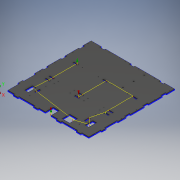
# Autodesk Inventor part: BA09
Saved by Autodesk Inventor 2017 (Build 210142000, 142)
## iProperties
Created: 2019-05-29
Part Number: BA09
Material: Wood (Cherry)
Document SubType Name: Modeling
Designer: Dell
Density: 0.63 g/cm^3
Appearance: Smooth - Black
Mass: 1071.87 g
Surface Area: 5591.98 cm^2
Volume: 1701.39 cm^3
Author: Dell
Autodesk Inventor part; units mm, degrees
(part 1 of 2)
ref_plane "YZ Plane" through (0, 0, 0) normal (1, 0, 0) x (0, 1, 0)
ref_plane "XZ Plane" through (0, 0, 0) normal (0, 1, 0) x (-1, 0, 0)
ref_plane "XY Plane" through (0, 0, 0) normal (0, 0, 1) x (1, 0, 0)
sketch "Sketch1" plane through (0, 0, 0) normal (0, 0, 1) x (1, 0, 0)
  line L0 (0, 0) -> (525.78, 0)
  line L1 (525.78, 0) -> (525.78, 355.6)
  line L2 (525.78, 355.6) -> (0, 355.6)
  line L3 (0, 355.6) -> (0, 0)
  dimension "d0" = 525.78
  dimension "d1" = 355.6
  constraints: 8 end point, 2 parallel, 1 horizontal, 1 perpendicular
  measures "d0" distance of L2.end L1.end
  measures "d1" distance of L2.end L0.start
extrude "Extrusion1" add sketch "Sketch1" along normal blind 6.35
sketch "Sketch2" plane through (0, 0, 6.35) normal (0, 0, 1) x (1, 0, 0)
  line L0 (525.78, 0) -> (525.78, 355.6) projected
  line L1 (525.78, 306.07) -> (518.16, 306.07)
  line L2 (518.16, 306.07) -> (518.16, 278.13)
  line L3 (518.16, 278.13) -> (525.78, 278.13)
  line L4 (525.78, 278.13) -> (525.78, 306.07)
  line L5 (525.78, 191.77) -> (518.16, 191.77)
  line L6 (518.16, 191.77) -> (518.16, 163.83)
  line L7 (518.16, 163.83) -> (525.78, 163.83)
  line L8 (525.78, 163.83) -> (525.78, 191.77)
  line L9 (525.78, 77.47) -> (518.16, 77.47)
  line L10 (518.16, 77.47) -> (518.16, 49.53)
  line L11 (518.16, 49.53) -> (525.78, 49.53)
  line L12 (525.78, 49.53) -> (525.78, 77.47)
  line L13 (0, 306.07) -> (7.62, 306.07)
  line L14 (7.62, 306.07) -> (7.62, 278.13)
  line L15 (7.62, 278.13) -> (0, 278.13)
  line L16 (0, 278.13) -> (0, 306.07)
  line L17 (0, 355.6) -> (0, 0) projected
  line L18 (0, 163.83) -> (7.62, 163.83)
  line L19 (7.62, 163.83) -> (7.62, 191.77)
  line L20 (7.62, 191.77) -> (0, 191.77)
  line L21 (0, 191.77) -> (0, 163.83)
  line L22 (0, 77.47) -> (7.62, 77.47)
  line L23 (7.62, 77.47) -> (7.62, 49.53)
  line L24 (7.62, 49.53) -> (0, 49.53)
  line L25 (0, 49.53) -> (0, 77.47)
  point P0 (0, 177.8)
  point P1 (525.78, 177.8)
  dimension "d4" = 7.62
  dimension "d5" = 7.62
  dimension "d6" = 27.94
  dimension "d7" = 27.94
  dimension "d8" = 27.94
  dimension "d9" = 49.53
  dimension "d10" = 49.53
  constraints: 48 end point, 12 parallel, 8 point on line, 6 horizontal, 6 perpendicular, 5 horizontal alignment, 4 midpoint, 4 vertical alignment
  measures "d4" distance of L13.start L13.end
  measures "d5" distance of L1.start L1.end
  measures "d6" distance of L13.end L14.end
  measures "d7" distance of L18.end L19.end
  measures "d8" distance of L22.end L23.end
  measures "d9" distance of L17.start L13.start
  measures "d10" distance of L17.end L24.end
extrude "Extrusion2" cut sketch "Sketch2" against normal through all
sketch "Sketch3" plane through (0, 0, 6.35) normal (0, 0, 1) x (1, 0, 0)
  line L0 (0, 0) -> (525.78, 0)
  line L1 (525.78, 0) -> (525.78, -184.15)
  line L2 (525.78, -184.15) -> (0, -184.15)
  line L3 (0, -184.15) -> (0, 0)
  line L4 (525.78, 355.6) -> (0, 355.6) projected
  line L5 (0, -78.105) -> (7.62, -78.105)
  line L6 (7.62, -78.105) -> (7.62, -106.045)
  line L7 (7.62, -106.045) -> (0, -106.045)
  line L8 (0, -106.045) -> (0, -78.105)
  line L9 (525.78, -78.105) -> (518.16, -78.105)
  line L10 (518.16, -78.105) -> (518.16, -106.045)
  line L11 (518.16, -106.045) -> (525.78, -106.045)
  line L12 (525.78, -106.045) -> (525.78, -78.105)
  line L13 (525.78, -79.375) -> (539.75, -79.375)
  line L14 (539.75, -79.375) -> (539.75, -104.775)
  line L15 (539.75, -104.775) -> (525.78, -104.775)
  line L16 (525.78, -104.775) -> (525.78, -79.375)
  line L17 (0, -79.375) -> (-13.97, -79.375)
  line L18 (-13.97, -79.375) -> (-13.97, -104.775)
  line L19 (-13.97, -104.775) -> (0, -104.775)
  line L20 (0, -104.775) -> (0, -79.375)
  point P0 (7.62, 49.53)
  point P1 (518.16, 49.53)
  point P2 (525.78, -92.075)
  point P3 (0, -92.075)
  dimension "d13" = 539.75
  dimension "d16" = 27.94
  dimension "d17" = 27.94
  dimension "d18" = 25.4
  dimension "d19" = 13.97
  dimension "d20" = 13.97
  dimension "d21" = 25.4
  constraints: 40 end point, 10 parallel, 6 midpoint, 5 horizontal, 5 perpendicular, 4 point on line, 2 vertical alignment, 1 coincident
  measures "d13" distance between parallel lines of L4 L2
  measures "d16" distance of L5.end L6.end
  measures "d17" distance of L9.end L10.end
  measures "d18" distance of L13.end L14.end
  measures "d19" distance of L13.start L13.end
  measures "d20" distance of L19.end L18.end
  measures "d21" distance of L18.end L17.end
extrude "Extrusion3" add sketch "Sketch3" against normal blind 6.35
sketch "Sketch4" plane through (0, 0, 6.35) normal (0, 0, 1) x (1, 0, 0)
  line L0 (525.78, 49.53) -> (525.78, -79.375) projected
  line L1 (525.78, -184.15) -> (0, -184.15) projected
  line L2 (525.78, 0) -> (518.16, 0)
  line L3 (518.16, 0) -> (518.16, -184.15)
  line L4 (518.16, -184.15) -> (525.78, -184.15)
  line L5 (525.78, -184.15) -> (525.78, 0)
  line L6 (525.78, -79.375) -> (539.75, -79.375) projected
  line L7 (525.78, -79.375) -> (518.16, -79.375)
  line L8 (518.16, -79.375) -> (518.16, -104.775)
  line L9 (518.16, -104.775) -> (525.78, -104.775)
  line L10 (525.78, -104.775) -> (525.78, -79.375)
  line L11 (0, 0) -> (7.62, 0)
  line L12 (7.62, 0) -> (7.62, -184.15)
  line L13 (7.62, -184.15) -> (0, -184.15)
  line L14 (0, -184.15) -> (0, 0)
  line L15 (0, -79.375) -> (7.62, -79.375)
  line L16 (7.62, -79.375) -> (7.62, -104.775)
  line L17 (7.62, -104.775) -> (0, -104.775)
  line L18 (0, -104.775) -> (0, -79.375)
  line L19 (525.78, -79.375) -> (539.75, -79.375)
  line L20 (539.75, -79.375) -> (539.75, -104.775)
  line L21 (539.75, -104.775) -> (525.78, -104.775)
  line L22 (525.78, -104.775) -> (525.78, -79.375)
  line L23 (0, -104.775) -> (-13.97, -104.775) projected
  line L24 (0, -104.775) -> (-13.97, -104.775)
  line L25 (-13.97, -104.775) -> (-13.97, -79.375)
  line L26 (-13.97, -79.375) -> (0, -79.375)
  line L27 (0, -79.375) -> (0, -104.775)
  line L28 (-13.97, -79.375) -> (-13.97, -104.775) projected
  point P0 (0, -104.775)
  point P1 (518.16, 49.53)
  point P2 (7.62, 49.53)
  constraints: 48 end point, 12 parallel, 8 point on line, 6 horizontal, 6 perpendicular, 2 coincident, 2 vertical alignment, 1 horizontal alignment
extrude "Extrusion4" cut sketch "Sketch4" against normal through all contours L0 L7 L3 L2 | L6 L20 L21 L5 | L5 L1 L3 L9 | L1 L14 L17 L12 | L23 L25 L26 L14 | L15 L14 L11 L12
sketch "Sketch5" plane through (0, 0, 6.35) normal (0, 0, 1) x (1, 0, 0)
  line L0 (518.16, -184.15) -> (7.62, -184.15) projected
  line L1 (518.16, -184.15) -> (518.16, -104.775) projected
  line L2 (7.62, -184.15) -> (518.16, -184.15)
  line L3 (518.16, -184.15) -> (518.16, -177.8)
  line L4 (518.16, -177.8) -> (7.62, -177.8)
  line L5 (7.62, -177.8) -> (7.62, -184.15)
  point P0 (0, 0)
  dimension "d24" = 6.35
  constraints: 8 end point, 2 parallel, 1 horizontal, 1 perpendicular, 1 point on line
  measures "d24" distance between parallel lines of L0 L4
extrude "Extrusion5" cut sketch "Sketch5" against normal through all
sketch "Sketch6" plane through (0, 0, 6.35) normal (0, 0, 1) x (1, 0, 0)
  line L0 (518.16, -177.8) -> (7.62, -177.8) projected
  line L1 (50.8, -177.8) -> (76.2, -177.8)
  line L2 (76.2, -177.8) -> (76.2, -185.42)
  line L3 (76.2, -185.42) -> (50.8, -185.42)
  line L4 (50.8, -185.42) -> (50.8, -177.8)
  line L5 (177.8, -177.8) -> (203.2, -177.8)
  line L6 (203.2, -177.8) -> (203.2, -185.42)
  line L7 (203.2, -185.42) -> (177.8, -185.42)
  line L8 (177.8, -185.42) -> (177.8, -177.8)
  line L9 (322.58, -177.8) -> (347.98, -177.8)
  line L10 (347.98, -177.8) -> (347.98, -185.42)
  line L11 (347.98, -185.42) -> (322.58, -185.42)
  line L12 (322.58, -185.42) -> (322.58, -177.8)
  line L13 (449.58, -177.8) -> (474.98, -177.8)
  line L14 (474.98, -177.8) -> (474.98, -185.42)
  line L15 (474.98, -185.42) -> (449.58, -185.42)
  line L16 (449.58, -185.42) -> (449.58, -177.8)
  line L17 (7.62, -104.775) -> (7.62, -177.8) projected
  line L18 (518.16, -177.8) -> (518.16, -104.775) projected
  line L19 (0, -79.375) -> (0, -104.775) projected
  line L20 (525.78, -104.775) -> (525.78, -79.375) projected
  point P0 (0, 0)
  dimension "d27" = 7.62
  dimension "d28" = 25.4
  dimension "d29" = 25.4
  dimension "d30" = 25.4
  dimension "d31" = 25.4
  dimension "d33" = 101.6
  dimension "d35" = 101.6
  dimension "d41" = 50.8
  dimension "d42" = 50.8
  constraints: 32 end point, 8 parallel, 6 point on line, 4 horizontal, 4 perpendicular, 1 horizontal alignment
  measures "d27" distance of L3.end L1.start
  measures "d28" distance of L2.end L3.end
  measures "d29" distance of L6.end L7.end
  measures "d30" distance of L10.end L11.end
  measures "d31" distance of L14.end L15.end
  measures "d33" distance between parallel lines of L2 L8
  measures "d35" distance between parallel lines of L16 L10
  measures "d41" distance from line of L19 L1.start
  measures "d42" distance from line of L20 L14.end
extrude "Extrusion6" add sketch "Sketch6" against normal blind 6.35
sketch "Sketch7" plane through (0, 0, 6.35) normal (0, 0, 1) x (1, 0, 0)
  line L0 (525.78, 355.6) -> (0, 355.6) projected
  line L1 (62.69, 355.6) -> (88.09, 355.6)
  line L2 (88.09, 355.6) -> (88.09, 347.98)
  line L3 (88.09, 347.98) -> (62.69, 347.98)
  line L4 (62.69, 347.98) -> (62.69, 355.6)
  line L5 (275.59, 355.6) -> (250.19, 355.6)
  line L6 (250.19, 355.6) -> (250.19, 347.98)
  line L7 (250.19, 347.98) -> (275.59, 347.98)
  line L8 (275.59, 347.98) -> (275.59, 355.6)
  line L9 (437.69, 355.6) -> (463.09, 355.6)
  line L10 (463.09, 355.6) -> (463.09, 347.98)
  line L11 (463.09, 347.98) -> (437.69, 347.98)
  line L12 (437.69, 347.98) -> (437.69, 355.6)
  line L13 (525.78, 355.6) -> (0, 355.6) projected
  line L14 (75.39, 347.98) -> (450.39, 347.98) construction
  point P0 (0, 0)
  point P1 (474.98, -185.42)
  point P2 (449.58, -185.42)
  point P3 (347.98, -185.42)
  point P4 (322.58, -185.42)
  point P5 (203.2, -185.42)
  point P6 (177.8, -185.42)
  point P7 (76.2, -185.42)
  point P8 (50.8, -185.42)
  point P9 (262.89, 355.6)
  point P10 (262.89, 347.98)
  point P11 (262.89, 355.6)
  dimension "d38" = 7.62
  dimension "d75" = 25.4
  dimension "d100" = 25.4
  dimension "d101" = 25.4
  dimension "d102" = 375
  constraints: 26 end point, 6 midpoint, 6 parallel, 3 horizontal, 3 horizontal alignment, 3 perpendicular, 3 point on line, 1 vertical alignment
  measures "d38" distance of L3.end L1.start
  measures "d75" distance of L6.end L7.end
  measures "d100" distance of L2.end L3.end
  measures "d101" distance of L10.end L11.end
  measures "d102" distance of L14.start L14.end
extrude "Extrusion7" cut sketch "Sketch7" against normal through all
sketch "Sketch8" plane through (0, 0, 6.35) normal (0, 0, 1) x (1, 0, 0)
  line L0 (242.89, -177.8) -> (282.89, -177.8)
  line L1 (282.89, -177.8) -> (282.89, -127.8)
  line L2 (282.89, -127.8) -> (242.89, -127.8)
  line L3 (242.89, -127.8) -> (242.89, -177.8)
  line L4 (203.2, -177.8) -> (322.58, -177.8) projected
  line L5 (518.16, -177.8) -> (518.16, -104.775) projected
  point P0 (0, 0)
  point P1 (262.89, -177.8)
  dimension "d43" = 50
  dimension "d44" = 40
  constraints: 8 end point, 2 midpoint, 2 parallel, 1 horizontal, 1 perpendicular, 1 point on line
  measures "d43" distance of L0.end L1.end
  measures "d44" distance of L1.end L2.end
extrude "Extrusion8" cut sketch "Sketch8" against normal through all
sketch "Sketch9" plane through (0, 0, 6.35) normal (0, 0, 1) x (1, 0, 0)
  line L0 (58.42, -76.2) -> (83.82, -76.2)
  line L1 (83.82, -76.2) -> (83.82, -127)
  line L2 (83.82, -127) -> (58.42, -127)
  line L3 (58.42, -127) -> (58.42, -76.2)
  line L4 (441.96, -127) -> (467.36, -127)
  line L5 (467.36, -127) -> (467.36, -76.2)
  line L6 (467.36, -76.2) -> (441.96, -76.2)
  line L7 (441.96, -76.2) -> (441.96, -127)
  line L8 (7.62, -104.775) -> (7.62, -177.8) projected
  line L9 (76.2, -177.8) -> (177.8, -177.8) projected
  line L10 (347.98, -177.8) -> (449.58, -177.8) projected
  line L11 (518.16, -177.8) -> (518.16, -104.775) projected
  point P0 (0, 0)
  dimension "d48" = 50.8
  dimension "d49" = 25.4
  dimension "d50" = 50.8
  dimension "d51" = 50.8
  dimension "d52" = 50.8
  dimension "d53" = 25.4
  dimension "d54" = 50.8
  dimension "d55" = 50.8
  constraints: 16 end point, 4 parallel, 2 horizontal, 2 perpendicular
  measures "d48" distance between parallel lines of L8 L3
  measures "d49" distance of L1.end L2.end
  measures "d50" distance of L2.end L0.start
  measures "d51" distance between parallel lines of L9 L2
  measures "d52" distance between parallel lines of L10 L4
  measures "d53" distance of L4.start L4.end
  measures "d54" distance of L6.end L4.start
  measures "d55" distance between parallel lines of L11 L5
extrude "Extrusion9" cut sketch "Sketch9" against normal through all
sketch "Sketch10" plane through (0, 0, 6.35) normal (0, 0, 1) x (1, 0, 0)
  line L0 (333.69, -114.3) -> (384.49, -114.3)
  line L1 (384.49, -114.3) -> (384.49, -165.1)
  line L2 (384.49, -165.1) -> (333.69, -165.1)
  line L3 (333.69, -165.1) -> (333.69, -114.3)
  line L4 (282.89, -127.8) -> (282.89, -177.8) projected
  line L5 (282.89, -177.8) -> (322.58, -177.8) projected
  point P0 (0, 0)
  point P1 (359.09, -165.1)
  dimension "d58" = 50.8
  dimension "d59" = 50.8
  dimension "d62" = 50.8
  dimension "d63" = 12.7
  constraints: 8 end point, 2 parallel, 1 horizontal, 1 midpoint, 1 perpendicular
  measures "d58" distance of L1.end L2.end
  measures "d59" distance of L0.end L1.end
  measures "d62" distance between parallel lines of L4 L3
  measures "d63" distance between parallel lines of L5 L2
extrude "Extrusion10" cut sketch "Sketch10" against normal through all
sketch "Sketch11" plane through (0, 0, 6.35) normal (0, 0, 1) x (1, 0, 0)
  line L0 (102.616, -101.6) -> (108.966, -101.6)
  line L1 (108.966, -101.6) -> (108.966, -76.2)
  line L2 (108.966, -76.2) -> (102.616, -76.2)
  line L3 (102.616, -76.2) -> (102.616, -101.6)
  line L4 (416.56, -101.6) -> (422.91, -101.6)
  line L5 (422.91, -101.6) -> (422.91, -76.2)
  line L6 (422.91, -76.2) -> (416.56, -76.2)
  line L7 (416.56, -76.2) -> (416.56, -101.6)
  line L8 (7.62, -104.775) -> (7.62, -177.8) projected
  line L9 (7.62, -177.8) -> (50.8, -177.8) projected
  line L10 (518.16, -177.8) -> (518.16, -104.775) projected
  line L11 (101.346, -74.93) -> (110.236, -74.93)
  line L12 (110.236, -74.93) -> (110.236, -102.87)
  line L13 (110.236, -102.87) -> (101.346, -102.87)
  line L14 (101.346, -102.87) -> (101.346, -74.93)
  line L15 (415.29, -74.93) -> (424.18, -74.93)
  line L16 (424.18, -74.93) -> (424.18, -102.87)
  line L17 (424.18, -102.87) -> (415.29, -102.87)
  line L18 (415.29, -102.87) -> (415.29, -74.93)
  point P0 (0, 0)
  point P1 (108.966, -88.9)
  point P2 (110.236, -88.9)
  point P3 (105.791, -76.2)
  point P4 (105.791, -74.93)
  point P5 (419.735, -76.2)
  point P6 (419.735, -74.93)
  point P7 (422.91, -88.9)
  point P8 (424.18, -88.9)
  dimension "d64" = 25.4
  dimension "d65" = 94.996
  dimension "d66" = 6.35
  dimension "d67" = 76.2
  dimension "d68" = 6.35
  dimension "d69" = 95.25
  dimension "d70" = 1.27
  dimension "d71" = 1.27
  dimension "d72" = 1.27
  constraints: 32 end point, 8 midpoint, 8 parallel, 4 horizontal, 4 horizontal alignment, 4 perpendicular, 2 vertical alignment, 1 point on line
  measures "d64" distance of L0.end L1.end
  measures "d65" distance between parallel lines of L8 L3
  measures "d66" distance of L1.end L2.end
  measures "d67" distance from line of L9 L0.end
  measures "d68" distance of L5.end L6.end
  measures "d69" distance between parallel lines of L10 L5
  measures "d70" distance between parallel lines of L15 L6
  measures "d71" distance between parallel lines of L16 L5
  measures "d72" distance between parallel lines of L1 L12
extrude "Extrusion11" cut sketch "Sketch11" against normal through all contours L3 L2 L1 L0 | L7 L6 L5 L4 | L11 L12 L13 L14 | L15 L16 L17 L18
sketch "Sketch12" plane through (0, 0, 6.35) normal (0, 0, 1) x (1, 0, 0)
  line L0 (62.69, 31.75) -> (88.09, 31.75)
  line L1 (88.09, 31.75) -> (88.09, 25.4)
  line L2 (88.09, 25.4) -> (62.69, 25.4)
  line L3 (62.69, 25.4) -> (62.69, 31.75)
  line L4 (250.19, 31.75) -> (275.59, 31.75)
  line L5 (275.59, 31.75) -> (275.59, 25.4)
  line L6 (275.59, 25.4) -> (250.19, 25.4)
  line L7 (250.19, 25.4) -> (250.19, 31.75)
  line L8 (437.69, 31.75) -> (463.09, 31.75)
  line L9 (463.09, 31.75) -> (463.09, 25.4)
  line L10 (463.09, 25.4) -> (437.69, 25.4)
  line L11 (437.69, 25.4) -> (437.69, 31.75)
  line L12 (7.62, -177.8) -> (50.8, -177.8) projected
  line L13 (0, 49.53) -> (0, 0) projected
  line L14 (525.78, 49.53) -> (525.78, 0) projected
  line L15 (88.09, 347.98) -> (62.69, 347.98) projected
  line L16 (275.59, 347.98) -> (250.19, 347.98) projected
  line L17 (463.09, 347.98) -> (437.69, 347.98) projected
  point P0 (88.09, 28.575)
  point P1 (250.19, 28.575)
  point P2 (75.39, 31.75)
  point P3 (75.39, 347.98)
  point P4 (262.89, 31.75)
  point P5 (262.89, 347.98)
  point P6 (450.39, 347.98)
  point P7 (450.39, 31.75)
  dimension "d77" = 6.35
  dimension "d78" = 25.4
  dimension "d79" = 25.4
  dimension "d81" = 25.4
  dimension "d82" = 203.2
  constraints: 24 end point, 8 midpoint, 6 parallel, 3 horizontal, 3 horizontal alignment, 3 perpendicular, 3 vertical alignment, 2 point on line
  measures "d77" distance of L2.end L0.start
  measures "d78" distance of L0.start L0.end
  measures "d79" distance of L4.start L4.end
  measures "d81" distance of L8.start L8.end
  measures "d82" distance between parallel lines of L12 L2
extrude "Extrusion12" cut sketch "Sketch12" against normal through all
sketch "Sketch13" plane through (0, 0, 6.35) normal (0, 0, 1) x (1, 0, 0)
  line L0 (62.69, 184.15) -> (88.09, 184.15)
  line L1 (88.09, 184.15) -> (88.09, 177.8)
  line L2 (88.09, 177.8) -> (62.69, 177.8)
  line L3 (62.69, 177.8) -> (62.69, 184.15)
  line L4 (250.19, 184.15) -> (275.59, 184.15)
  line L5 (275.59, 184.15) -> (275.59, 177.8)
  line L6 (275.59, 177.8) -> (250.19, 177.8)
  line L7 (250.19, 177.8) -> (250.19, 184.15)
  line L8 (463.09, 177.8) -> (437.69, 177.8)
  line L9 (437.69, 177.8) -> (437.69, 184.15)
  line L10 (437.69, 184.15) -> (463.09, 184.15)
  line L11 (463.09, 184.15) -> (463.09, 177.8)
  line L12 (88.09, 347.98) -> (62.69, 347.98) projected
  line L13 (275.59, 347.98) -> (250.19, 347.98) projected
  line L14 (463.09, 347.98) -> (437.69, 347.98) projected
  line L15 (62.69, 355.6) -> (0, 355.6) projected
  point P0 (0, 0)
  point P1 (75.39, 184.15)
  point P2 (75.39, 347.98)
  point P3 (262.89, 184.15)
  point P4 (262.89, 347.98)
  point P5 (450.39, 184.15)
  point P6 (450.39, 347.98)
  point P7 (262.89, 347.98)
  point P8 (450.39, 347.98)
  dimension "d89" = 25.4
  dimension "d90" = 6.35
  dimension "d93" = 25.4
  dimension "d94" = 6.35
  dimension "d95" = 25.4
  dimension "d96" = 6.35
  dimension "d97" = 177.8
  constraints: 24 end point, 8 midpoint, 6 parallel, 5 vertical alignment, 3 horizontal, 3 perpendicular, 2 horizontal alignment
  measures "d89" distance of L1.end L2.end
  measures "d90" distance of L0.end L1.end
  measures "d93" distance of L5.end L6.end
  measures "d94" distance of L4.end L5.end
  measures "d95" distance of L9.end L10.end
  measures "d96" distance of L8.end L9.end
  measures "d97" distance between parallel lines of L2 L15
extrude "Extrusion13" cut sketch "Sketch13" against normal through all
sketch "Sketch14" plane through (0, 0, 6.35) normal (0, 0, 1) x (1, 0, 0)
  line L0 (62.69, 6.35) -> (88.09, 6.35)
  line L1 (88.09, 6.35) -> (88.09, 0)
  line L2 (88.09, 0) -> (62.69, 0)
  line L3 (62.69, 0) -> (62.69, 6.35)
  line L4 (250.19, 6.35) -> (275.59, 6.35)
  line L5 (275.59, 6.35) -> (275.59, 0)
  line L6 (275.59, 0) -> (250.19, 0)
  line L7 (250.19, 0) -> (250.19, 6.35)
  line L8 (437.69, 6.35) -> (463.09, 6.35)
  line L9 (463.09, 6.35) -> (463.09, 0)
  line L10 (463.09, 0) -> (437.69, 0)
  line L11 (437.69, 0) -> (437.69, 6.35)
  line L12 (7.62, -177.8) -> (50.8, -177.8) projected
  point P0 (0, 0)
  point P1 (88.09, 25.4)
  point P2 (62.69, 25.4)
  point P3 (250.19, 25.4)
  point P4 (275.59, 25.4)
  point P5 (437.69, 25.4)
  point P6 (463.09, 25.4)
  dimension "d103" = 184.15
  dimension "d104" = 6.35
  constraints: 24 end point, 6 parallel, 6 vertical alignment, 3 horizontal, 3 horizontal alignment, 3 perpendicular, 2 point on line
  measures "d103" distance between parallel lines of L12 L0
  measures "d104" distance of L2.end L0.start
extrude "Extrusion14" cut sketch "Sketch14" against normal through all
sketch "Sketch15" plane through (0, 0, 6.35) normal (0, 0, 1) x (1, 0, 0)
  circle A0 centre (118.34, 352.425) radius 2.25
  circle A1 centre (219.94, 352.425) radius 2.25
  circle A2 centre (305.84, 352.425) radius 2.25
  circle A3 centre (407.44, 352.425) radius 2.25
  line L0 (250.19, 355.6) -> (88.09, 355.6) projected
  line L1 (75.39, 352.425) -> (118.34, 352.425)
  line L2 (219.94, 352.425) -> (262.89, 352.425)
  line L3 (262.89, 352.425) -> (305.84, 352.425)
  line L4 (88.09, 347.98) -> (62.69, 347.98) projected
  line L5 (275.59, 347.98) -> (250.19, 347.98) projected
  line L6 (407.44, 352.425) -> (450.39, 352.425)
  line L7 (463.09, 347.98) -> (437.69, 347.98) projected
  circle A4 centre (118.34, 180.975) radius 2.25
  circle A5 centre (219.94, 180.975) radius 2.25
  circle A6 centre (305.84, 180.975) radius 2.25
  circle A7 centre (407.44, 180.975) radius 2.25
  line L8 (88.09, 184.15) -> (88.09, 177.8) projected
  circle A8 centre (118.34, 28.575) radius 2.25
  circle A9 centre (219.94, 28.575) radius 2.25
  circle A10 centre (305.84, 28.575) radius 2.25
  circle A11 centre (407.44, 28.575) radius 2.25
  circle A12 centre (118.34, 3.175) radius 2.25
  circle A13 centre (219.94, 3.175) radius 2.25
  circle A14 centre (305.84, 3.175) radius 2.25
  circle A15 centre (407.44, 3.175) radius 2.25
  line L9 (88.09, 31.75) -> (88.09, 25.4) projected
  line L10 (88.09, 6.35) -> (88.09, 0) projected
  circle A16 centre (105.791, -38.1) radius 2.25
  circle A17 centre (105.791, -139.7) radius 2.25
  circle A18 centre (419.735, -38.1) radius 2.25
  circle A19 centre (419.735, -139.7) radius 2.25
  line L11 (101.346, -74.93) -> (110.236, -74.93) projected
  line L12 (415.29, -74.93) -> (424.18, -74.93) projected
  line L13 (105.791, -38.1) -> (105.791, -139.7) construction
  line L14 (419.735, -38.1) -> (419.735, -139.7) construction
  line L15 (110.236, -74.93) -> (110.236, -102.87) projected
  line L16 (415.29, -102.87) -> (415.29, -74.93) projected
  circle A20 centre (3.81, 24.765) radius 2.25
  circle A21 centre (3.81, 120.65) radius 2.25
  circle A22 centre (3.81, 234.95) radius 2.25
  circle A23 centre (3.81, 330.835) radius 2.25
  line L17 (0, 0) -> (7.62, 0) projected
  line L18 (0, 355.6) -> (0, 306.07) projected
  line L19 (0, 278.13) -> (0, 191.77) projected
  line L20 (0, 163.83) -> (0, 77.47) projected
  line L21 (0, 49.53) -> (0, 0) projected
  line L22 (282.89, -127.8) -> (242.89, -127.8) projected
  line L23 (262.89, -127.8) -> (262.89, -65.7768)
  circle A24 centre (521.97, 24.765) radius 2.25
  circle A25 centre (521.97, 120.65) radius 2.25
  circle A26 centre (521.97, 234.95) radius 2.25
  circle A27 centre (521.97, 330.835) radius 2.25
  line L24 (525.78, 0) -> (518.16, 0)
  line L25 (525.78, 355.6) -> (525.78, 306.07)
  line L26 (525.78, 278.13) -> (525.78, 191.77)
  line L27 (525.78, 163.83) -> (525.78, 77.47)
  line L28 (525.78, 49.53) -> (525.78, 0)
  point P0 (75.39, 347.98)
  point P1 (262.89, 347.98)
  point P2 (450.39, 347.98)
  point P3 (88.09, 180.975)
  point P4 (88.09, 28.575)
  point P5 (88.09, 3.175)
  point P6 (105.791, -74.93)
  point P7 (419.735, -74.93)
  point P8 (105.791, -88.9)
  point P9 (110.236, -88.9)
  point P10 (419.735, -88.9)
  point P11 (415.29, -88.9)
  point P12 (3.81, 0)
  point P13 (0, 330.835)
  point P14 (0, 234.95)
  point P15 (0, 120.65)
  point P16 (0, 24.765)
  point P17 (3.81, 0)
  point P18 (521.97, 0)
  point P19 (525.78, 330.835)
  point P20 (525.78, 234.95)
  point P21 (525.78, 120.65)
  point P22 (525.78, 24.765)
  point P23 (521.97, 0)
  dimension "d107" = 4.5
  dimension "d108" = 4.5
  dimension "d109" = 4.5
  dimension "d110" = 4.5
  dimension "d111" = 3.175
  dimension "d112" = 42.95
  dimension "d113" = 42.95
  dimension "d114" = 42.95
  dimension "d115" = 42.95
  dimension "d116" = 4.5
  dimension "d117" = 4.5
  dimension "d118" = 4.5
  dimension "d119" = 4.5
  dimension "d120" = 4.5
  dimension "d121" = 4.5
  dimension "d122" = 4.5
  dimension "d123" = 4.5
  dimension "d124" = 4.5
  dimension "d125" = 4.5
  dimension "d126" = 4.5
  dimension "d127" = 4.5
  dimension "d134" = 4.5
  dimension "d135" = 4.5
  dimension "d136" = 4.5
  dimension "d137" = 4.5
  dimension "d138" = 101.6
  dimension "d139" = 4.5
  dimension "d140" = 4.5
  dimension "d141" = 4.5
  dimension "d142" = 4.5
  constraints: 28 centre point, 24 end point, 23 vertical alignment, 22 horizontal alignment, 19 midpoint, 19 symmetric about line, 3 horizontal, 3 vertical, 1 collinear, 4 other
  measures "d107" diameter of A0
  measures "d108" diameter of A1
  measures "d109" diameter of A2
  measures "d110" diameter of A3
  measures "d111" distance from line of L0 L1.end
  measures "d112" distance of L1.start L1.end
  measures "d113" distance of L2.start L2.end
  measures "d114" distance of L2.end L3.end
  measures "d115" distance of L6.start L6.end
  measures "d116" diameter of A4
  measures "d117" diameter of A5
  measures "d118" diameter of A6
  measures "d119" diameter of A7
  measures "d120" diameter of A8
  measures "d121" diameter of A9
  measures "d122" diameter of A10
  measures "d123" diameter of A11
  measures "d124" diameter of A12
  measures "d125" diameter of A13
  measures "d126" diameter of A14
  measures "d127" diameter of A15
  measures "d134" diameter of A16
  measures "d135" diameter of A17
  measures "d136" diameter of A18
  measures "d137" diameter of A19
  measures "d138" distance of L14.start L14.end
  measures "d139" diameter of A20
  measures "d140" diameter of A21
  measures "d141" diameter of A22
  measures "d142" diameter of A23
extrude "Extrusion15" cut sketch "Sketch15" against normal through all
sketch "Sketch16" plane through (0, 0, 6.35) normal (0, 0, 1) x (1, 0, 0)
  circle A0 centre (356.64, 335.6) radius 4
  circle A1 centre (356.64, 267.89) radius 4
  circle A2 centre (356.64, 200.18) radius 4
  line L0 (437.69, 355.6) -> (275.59, 355.6) projected
  point P0 (0, 0)
  point P1 (356.64, 355.6)
  point P2 (356.64, 355.6)
  dimension "d145" = 8
  dimension "d146" = 8
  dimension "d147" = 8
  dimension "d148" = 20
  dimension "d149" = 67.71
  dimension "d150" = 67.71
  constraints: 3 centre point, 3 vertical alignment, 2 midpoint
  measures "d145" diameter of A0
  measures "d146" diameter of A1
  measures "d147" diameter of A2
  measures "d148" distance from line of L0 A0.centre
  measures "d149" distance of A0.centre A1.centre
  measures "d150" distance of A1.centre A2.centre
extrude "Extrusion16" cut sketch "Sketch16" against normal through all
sketch "Sketch17" plane through (0, 0, 6.35) normal (0, 0, 1) x (1, 0, 0)
  line L0 (62.69, 355.6) -> (0, 355.6) projected
  line L1 (61.42, 355.6) -> (89.36, 355.6)
  line L2 (89.36, 355.6) -> (89.36, 347.98)
  line L3 (89.36, 347.98) -> (61.42, 347.98)
  line L4 (61.42, 347.98) -> (61.42, 355.6)
  line L5 (250.19, 355.6) -> (88.09, 355.6) projected
  line L6 (248.92, 355.6) -> (276.86, 355.6)
  line L7 (276.86, 355.6) -> (276.86, 347.98)
  line L8 (276.86, 347.98) -> (248.92, 347.98)
  line L9 (248.92, 347.98) -> (248.92, 355.6)
  line L10 (437.69, 355.6) -> (275.59, 355.6) projected
  line L11 (436.42, 355.6) -> (464.36, 355.6)
  line L12 (464.36, 355.6) -> (464.36, 347.98)
  line L13 (464.36, 347.98) -> (436.42, 347.98)
  line L14 (436.42, 347.98) -> (436.42, 355.6)
  line L15 (62.69, 347.98) -> (62.69, 355.6) projected
  line L16 (88.09, 355.6) -> (88.09, 347.98) projected
  line L17 (250.19, 347.98) -> (250.19, 355.6) projected
  line L18 (275.59, 355.6) -> (275.59, 347.98) projected
  line L19 (437.69, 347.98) -> (437.69, 355.6) projected
  line L20 (463.09, 355.6) -> (463.09, 347.98) projected
  line L21 (61.42, 185.42) -> (89.36, 185.42)
  line L22 (89.36, 185.42) -> (89.36, 176.53)
  line L23 (89.36, 176.53) -> (61.42, 176.53)
  line L24 (61.42, 176.53) -> (61.42, 185.42)
  line L25 (62.69, 184.15) -> (88.09, 184.15) projected
  line L26 (62.69, 177.8) -> (62.69, 184.15) projected
  line L27 (248.92, 185.42) -> (276.86, 185.42)
  line L28 (276.86, 185.42) -> (276.86, 176.53)
  line L29 (276.86, 176.53) -> (248.92, 176.53)
  line L30 (248.92, 176.53) -> (248.92, 185.42)
  line L31 (250.19, 184.15) -> (275.59, 184.15) projected
  line L32 (250.19, 177.8) -> (250.19, 184.15) projected
  line L33 (436.42, 185.42) -> (464.36, 185.42)
  line L34 (464.36, 185.42) -> (464.36, 176.53)
  line L35 (464.36, 176.53) -> (436.42, 176.53)
  line L36 (436.42, 176.53) -> (436.42, 185.42)
  line L37 (61.42, 33.02) -> (89.36, 33.02)
  line L38 (89.36, 33.02) -> (89.36, 24.13)
  line L39 (89.36, 24.13) -> (61.42, 24.13)
  line L40 (61.42, 24.13) -> (61.42, 33.02)
  line L41 (248.92, 33.02) -> (276.86, 33.02)
  line L42 (276.86, 33.02) -> (276.86, 24.13)
  line L43 (276.86, 24.13) -> (248.92, 24.13)
  line L44 (248.92, 24.13) -> (248.92, 33.02)
  line L45 (436.42, 33.02) -> (464.36, 33.02)
  line L46 (464.36, 33.02) -> (464.36, 24.13)
  line L47 (464.36, 24.13) -> (436.42, 24.13)
  line L48 (436.42, 24.13) -> (436.42, 33.02)
  line L49 (464.36, -1.27) -> (436.42, -1.27)
  line L50 (436.42, -1.27) -> (436.42, 7.62)
  line L51 (436.42, 7.62) -> (464.36, 7.62)
  line L52 (464.36, 7.62) -> (464.36, -1.27)
  line L53 (276.86, -1.27) -> (248.92, -1.27)
  line L54 (248.92, -1.27) -> (248.92, 7.62)
  line L55 (248.92, 7.62) -> (276.86, 7.62)
  line L56 (276.86, 7.62) -> (276.86, -1.27)
  line L57 (89.36, -1.27) -> (61.42, -1.27)
  line L58 (61.42, -1.27) -> (61.42, 7.62)
  line L59 (61.42, 7.62) -> (89.36, 7.62)
  line L60 (89.36, 7.62) -> (89.36, -1.27)
  line L61 (88.09, 31.75) -> (88.09, 25.4) projected
  line L62 (250.19, 25.4) -> (250.19, 31.75) projected
  line L63 (437.69, 25.4) -> (437.69, 31.75) projected
  line L64 (437.69, 184.15) -> (463.09, 184.15) projected
  line L65 (437.69, 177.8) -> (437.69, 184.15) projected
  line L66 (62.69, 31.75) -> (88.09, 31.75) projected
  line L67 (250.19, 31.75) -> (275.59, 31.75) projected
  line L68 (437.69, 31.75) -> (463.09, 31.75) projected
  line L69 (62.69, 6.35) -> (88.09, 6.35) projected
  line L70 (88.09, 6.35) -> (88.09, 0) projected
  line L71 (250.19, 0) -> (250.19, 6.35) projected
  line L72 (437.69, 0) -> (437.69, 6.35) projected
  line L73 (250.19, 6.35) -> (275.59, 6.35) projected
  line L74 (437.69, 6.35) -> (463.09, 6.35) projected
  line L75 (100.076, -73.66) -> (111.506, -73.66)
  line L76 (111.506, -73.66) -> (111.506, -104.14)
  line L77 (111.506, -104.14) -> (100.076, -104.14)
  line L78 (100.076, -104.14) -> (100.076, -73.66)
  line L79 (414.02, -73.66) -> (425.45, -73.66)
  line L80 (425.45, -73.66) -> (425.45, -104.14)
  line L81 (425.45, -104.14) -> (414.02, -104.14)
  line L82 (414.02, -104.14) -> (414.02, -73.66)
  line L83 (101.346, -74.93) -> (110.236, -74.93) projected
  line L84 (415.29, -74.93) -> (424.18, -74.93) projected
  line L85 (101.346, -102.87) -> (101.346, -74.93) projected
  line L86 (415.29, -102.87) -> (415.29, -74.93) projected
  line L87 (0, 307.34) -> (7.62, 307.34)
  line L88 (7.62, 307.34) -> (7.62, 276.86)
  line L89 (7.62, 276.86) -> (0, 276.86)
  line L90 (0, 276.86) -> (0, 307.34)
  line L91 (0, 355.6) -> (0, 306.07) projected
  line L92 (0, 306.07) -> (7.62, 306.07) projected
  line L93 (7.62, 306.07) -> (7.62, 278.13) projected
  line L94 (7.62, 278.13) -> (0, 278.13) projected
  line L95 (0, 278.13) -> (0, 191.77) projected
  line L96 (0, 193.04) -> (7.62, 193.04)
  line L97 (7.62, 193.04) -> (7.62, 162.56)
  line L98 (7.62, 162.56) -> (0, 162.56)
  line L99 (0, 162.56) -> (0, 193.04)
  line L100 (0, 163.83) -> (0, 77.47) projected
  line L101 (0, 78.74) -> (7.62, 78.74)
  line L102 (7.62, 78.74) -> (7.62, 48.26)
  line L103 (7.62, 48.26) -> (0, 48.26)
  line L104 (0, 48.26) -> (0, 78.74)
  line L105 (0, 191.77) -> (7.62, 191.77) projected
  line L106 (7.62, 163.83) -> (0, 163.83) projected
  line L107 (7.62, 77.47) -> (0, 77.47) projected
  line L108 (7.62, 49.53) -> (0, 49.53) projected
  line L109 (7.62, 77.47) -> (7.62, 49.53) projected
  line L110 (262.89, 185.42) -> (262.89, 243.6528)
  line L111 (525.78, 307.34) -> (518.16, 307.34)
  line L112 (518.16, 307.34) -> (518.16, 276.86)
  line L113 (518.16, 276.86) -> (525.78, 276.86)
  line L114 (525.78, 276.86) -> (525.78, 307.34)
  line L115 (525.78, 355.6) -> (525.78, 306.07)
  line L116 (525.78, 306.07) -> (518.16, 306.07)
  line L117 (518.16, 306.07) -> (518.16, 278.13)
  line L118 (518.16, 278.13) -> (525.78, 278.13)
  line L119 (525.78, 278.13) -> (525.78, 191.77)
  line L120 (525.78, 193.04) -> (518.16, 193.04)
  line L121 (518.16, 193.04) -> (518.16, 162.56)
  line L122 (518.16, 162.56) -> (525.78, 162.56)
  line L123 (525.78, 162.56) -> (525.78, 193.04)
  line L124 (525.78, 163.83) -> (525.78, 77.47)
  line L125 (525.78, 78.74) -> (518.16, 78.74)
  line L126 (518.16, 78.74) -> (518.16, 48.26)
  line L127 (518.16, 48.26) -> (525.78, 48.26)
  line L128 (525.78, 48.26) -> (525.78, 78.74)
  line L129 (525.78, 191.77) -> (518.16, 191.77)
  line L130 (518.16, 163.83) -> (525.78, 163.83)
  line L131 (518.16, 77.47) -> (525.78, 77.47)
  line L132 (518.16, 49.53) -> (525.78, 49.53)
  line L133 (518.16, 77.47) -> (518.16, 49.53)
  point P0 (0, 0)
  point P1 (75.39, 184.15)
  point P2 (75.39, 185.42)
  point P3 (62.69, 180.975)
  point P4 (61.42, 180.975)
  point P5 (262.89, 184.15)
  point P6 (250.19, 180.975)
  point P7 (248.92, 180.975)
  point P8 (88.09, 28.575)
  point P9 (89.36, 28.575)
  point P10 (248.92, 28.575)
  point P11 (250.19, 28.575)
  point P12 (437.69, 28.575)
  point P13 (436.42, 28.575)
  point P14 (437.69, 28.575)
  point P15 (450.39, 184.15)
  point P16 (450.39, 185.42)
  point P17 (437.69, 180.975)
  point P18 (436.42, 180.975)
  point P19 (75.39, 31.75)
  point P20 (75.39, 33.02)
  point P21 (262.89, 31.75)
  point P22 (262.89, 33.02)
  point P23 (450.39, 31.75)
  point P24 (450.39, 33.02)
  point P25 (88.09, 3.175)
  point P26 (89.36, 3.175)
  point P27 (250.19, 3.175)
  point P28 (248.92, 3.175)
  point P29 (437.69, 3.175)
  point P30 (436.42, 3.175)
  point P31 (262.89, 6.35)
  point P32 (262.89, 7.62)
  point P33 (450.39, 6.35)
  point P34 (450.39, 7.62)
  point P35 (75.39, 6.35)
  point P36 (75.39, 7.62)
  point P37 (105.791, -74.93)
  point P38 (105.791, -73.66)
  point P39 (419.735, -74.93)
  point P40 (419.735, -73.66)
  point P41 (101.346, -88.9)
  point P42 (100.076, -88.9)
  point P43 (415.29, -88.9)
  point P44 (414.02, -88.9)
  point P45 (7.62, 63.5)
  point P46 (525.78, 0)
  point P47 (518.16, 63.5)
  dimension "d153" = 1.27
  dimension "d154" = 1.27
  dimension "d155" = 1.27
  dimension "d156" = 1.27
  dimension "d157" = 1.27
  dimension "d158" = 1.27
  dimension "d159" = 1.27
  dimension "d161" = 1.27
  dimension "d162" = 1.27
  dimension "d163" = 1.27
  dimension "d164" = 1.27
  dimension "d165" = 1.27
  dimension "d166" = 1.27
  dimension "d167" = 1.27
  dimension "d168" = 1.27
  dimension "d169" = 1.27
  dimension "d170" = 1.27
  dimension "d171" = 1.27
  constraints: 184 end point, 48 midpoint, 34 parallel, 27 symmetric about line, 24 point on line, 20 vertical alignment, 17 horizontal, 17 perpendicular, 16 horizontal alignment, 1 vertical
  measures "d153" distance between parallel lines of L4 L15
  measures "d154" distance between parallel lines of L2 L16
  measures "d155" distance between parallel lines of L17 L9
  measures "d156" distance between parallel lines of L18 L7
  measures "d157" distance between parallel lines of L19 L14
  measures "d158" distance between parallel lines of L12 L20
  measures "d159" distance between parallel lines of L21 L25
  measures "d161" distance between parallel lines of L37 L66
  measures "d162" distance between parallel lines of L59 L69
  measures "d163" distance between parallel lines of L78 L85
  measures "d164" distance between parallel lines of L75 L83
  measures "d165" distance between parallel lines of L82 L86
  measures "d166" distance between parallel lines of L87 L92
  measures "d167" distance between parallel lines of L94 L89
  measures "d168" distance between parallel lines of L96 L105
  measures "d169" distance between parallel lines of L98 L106
  measures "d170" distance between parallel lines of L107 L101
  measures "d171" distance between parallel lines of L108 L103
extrude "Extrusion17" cut sketch "Sketch17" against normal through all